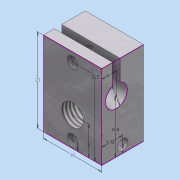
# Autodesk Inventor part: Chimera Heatblock
Saved by Autodesk Inventor 2016 (Build 200138000, 138)
## iProperties
Created: 2016-08-02
Part Number: Chimera Heatblock
Material: Aluminum 6061, Welded
Document SubType Name: Modeling
Designer: Sam
Density: 2.7 g/cm^3
Appearance: Weld - Aluminum
Author: Sam
Autodesk Inventor part; units mm, degrees
ref_plane "YZ Plane" through (0, 0, 0) normal (1, 0, 0) x (0, 1, 0)
ref_plane "XZ Plane" through (0, 0, 0) normal (0, 1, 0) x (-1, 0, 0)
ref_plane "XY Plane" through (0, 0, 0) normal (0, 0, 1) x (1, 0, 0)
sketch "Sketch1" plane through (0, 0, 0) normal (0, 1, 0) x (-1, 0, 0)
  line L0 (-6, 7) -> (10, 7)
  line L1 (10, 7) -> (10, -16)
  line L2 (10, -16) -> (-6, -16)
  line L3 (-6, -16) -> (-6, 7)
  point P0 (0, 0)
  point P1 (2, -8)
  point P2 (2, -14)
  point P3 (2, 4.5)
  dimension "d0" = 16
  dimension "d1" = 23
  dimension "d3" = 8
  dimension "d4" = 2
  dimension "d5" = 20.5
  constraints: 8 end point, 2 parallel, 1 horizontal, 1 perpendicular
  measures "d0" distance of L1.end L2.end
  measures "d1" distance of L0.end L1.end
  measures "d3" distance from line of L2 point (2, -8)
  measures "d4" distance from line of L2 point (2, -14)
  measures "d5" distance from line of point (2, 4.5) L2
extrude "Extrusion1" add sketch "Sketch1" along normal blind 11.5
hole "Hole1" at (-2, 0, -8) direction (0, 1, 0) diameter 6 end through all
hole "Hole2" at (-2, 0, 4.5) direction (0, 1, 0) diameter 3 end through all
hole "Hole3" at (-2, 0, -14) direction (0, 1, 0) diameter 3 depth 6 tip angle 118
sketch "Sketch3" plane through (6, 0, 7) normal (1, 0, 0) x (0, 0, -1)
  arc A0 (5.6761, 2.9874) -> (5.6761, 5.0126) centre (8.5, 4) ccw
  line L0 (23, 0) -> (0, 0)
  line L1 (23, 0) -> (23, 11.5)
  line L2 (0, 0) -> (0, 11.5)
  line L3 (5.6761, 5.0126) -> (0, 5.0126)
  line L4 (5.6761, 2.9874) -> (0, 2.9874)
  line L5 (0, 5.0126) -> (0, 2.9874)
  point P0 (16, 0)
  point P1 (21, 5.75)
  dimension "d29" = 6
  dimension "d30" = 4
  dimension "d31" = 14.5
  dimension "d32" = 2
  dimension "d33" = 5.75
  constraints: 12 end point, 3 perpendicular, 2 point on circle, 2 point on line, 1 centre point
  measures "d29" diameter of A0
  measures "d30" distance from line of L0 A0.centre
  measures "d31" distance from line of L1 A0.centre
  measures "d32" distance from line of L1 point (21, 5.75)
  measures "d33" distance from line of L0 point (21, 5.75)
extrude "Extrusion2" cut sketch "Sketch3" against normal blind 20
hole "Hole4" at (6, 5.75, -14) direction (-1, 0, 0) diameter 3 end through all
thread "Thread1" size "M3x0.5" class "6H" standard "ANSI Metric M Profile" full length
thread "Thread2" size "M3x0.5" class "6H" standard "ANSI Metric M Profile" full length
thread "Thread3" size "M3x0.5" class "6H" standard "ANSI Metric M Profile" full length
thread "Thread4" size "M6x1" class "6H" standard "ANSI Metric M Profile" full length
body "Solid1"
